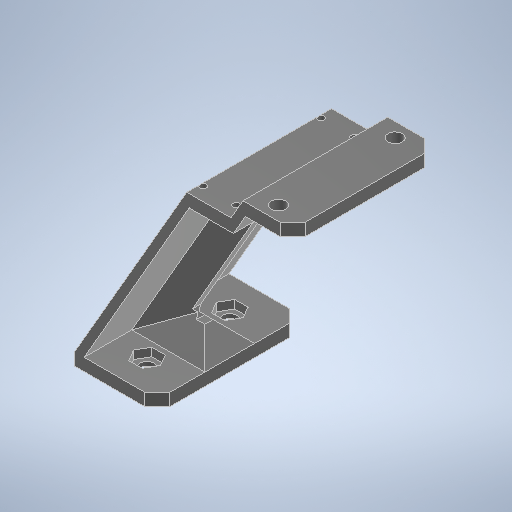
# Autodesk Inventor part: 3D_camera-fix
Saved by Autodesk Inventor 2025 (Build 290162000, 162)
## iProperties
Created: 2024-06-30
Part Number: 3D_camera-fix
Material: 一般
Document SubType Name: Modeling
Designer: 8326d
Density: 1 g/cm^3
Appearance: 滑らか - 黒
Author: 8326d
Autodesk Inventor part; units mm, degrees
ref_plane "YZ Plane" through (0, 0, 0) normal (1, 0, 0) x (0, 1, 0)
ref_plane "XZ Plane" through (0, 0, 0) normal (0, 1, 0) x (-1, 0, 0)
ref_plane "XY Plane" through (0, 0, 0) normal (0, 0, 1) x (1, 0, 0)
sketch "スケッチ1" plane through (0, 0, 0) normal (0, 0, 1) x (1, 0, 0)
  line L0 (120.5, 0) -> (-120.5, 0) construction
  line L1 (120.5, 0) -> (361.5, 0) construction
  line L2 (-120.5, 0) -> (-100.5, 0)
  line L3 (-100.5, 0) -> (-100.5, 3)
  line L4 (-100.5, 3) -> (-120.5, 3)
  line L5 (-120.5, 3) -> (-120.5, 0)
  line L6 (-120.5, 3) -> (-90.5, 54.961524) construction
  line L7 (-120.5, 3) -> (-60.5, 3) construction
  line L8 (-79.8, 54.961524) -> (-67.8, 54.961524)
  line L9 (-67.8, 54.961524) -> (-67.8, 51.961524)
  line L10 (-67.8, 51.961524) -> (-79.8, 51.961524)
  line L11 (-79.8, 51.961524) -> (-79.8, 54.961524)
  line L12 (-118.190599, 3) -> (-89.92265, 51.961524) construction
  line L13 (-118.190599, 3) -> (-92.809401, 46.961524)
  line L14 (-92.809401, 46.961524) -> (-82.109401, 46.961524)
  line L15 (-82.109401, 46.961524) -> (-79.22265, 51.961524)
  line L16 (-79.8, 54.961524) -> (-82.686751, 49.961524)
  line L17 (-82.686751, 49.961524) -> (-93.386751, 49.961524)
  line L18 (-93.386751, 49.961524) -> (-120.5, 3)
  point P0 (0, 0)
  point P1 (0, 0)
  point P2 (-118.190599, 3)
  dimension "d0" = 241
  dimension "d1" = 180
  dimension "d2" = 20
  dimension "d3" = 3
  dimension "d4" = 60
  dimension "d5" = 60
  dimension "d6" = 12
  dimension "d7" = 3
  dimension "d8" = 2
  dimension "d72" = 2
  dimension "d74" = 3
  dimension "d75" = 40.7
  dimension "d89" = 5
  constraints: 38 end point, 8 parallel, 6 horizontal, 3 point on line, 2 collinear, 2 equal length, 2 perpendicular, 1 coincident, 1 horizontal alignment, 1 midpoint
  measures "d0" distance of L0.start L0.end
  measures "d1" angle of L0 L1
  measures "d2" distance of L4.end L3.end
  measures "d3" distance of L3.end L2.end
  measures "d4" distance of L6.end L4.end
  measures "d5" angle of L7 L6
  measures "d6" distance of L9.end L10.end
  measures "d7" distance of L8.end L9.end
  measures "d8" distance between parallel lines of L6 L12
  measures "d72" distance between parallel lines of L16 L15
  measures "d74" distance between parallel lines of L14 L17
  measures "d75" distance between parallel lines of L5 L11
  measures "d89" distance between parallel lines of L8 L17
extrude "押し出し1" add sketch "スケッチ1" along normal mid plane 35
sketch "スケッチ2" plane through (0, 0, 0) normal (0, 0, 1) x (1, 0, 0)
  line L0 (-100.5, 3) -> (-120.5, 3)
  line L1 (-100.5, 3) -> (-105.5, 8)
  line L2 (-105.5, 8) -> (-109.530345, 8)
  line L3 (-76.335898, 46.961524) -> (-72.8, 46.961524)
  line L4 (-72.8, 46.961524) -> (-67.8, 51.961524)
  line L5 (-79.22265, 51.961524) -> (-82.109401, 46.961524)
  line L6 (-82.109401, 46.961524) -> (-92.809401, 46.961524)
  line L7 (-92.809401, 46.961524) -> (-118.190599, 3)
  line L8 (-76.335898, 46.961524) -> (-79.22265, 41.961524)
  line L9 (-79.22265, 41.961524) -> (-89.92265, 41.961524)
  line L10 (-89.92265, 41.961524) -> (-109.530345, 8)
  line L11 (-67.8, 51.961524) -> (-79.22265, 51.961524)
  point P0 (0, 0)
  dimension "d13" = 5
  dimension "d14" = 45
  dimension "d76" = 5
  dimension "d77" = 45
  dimension "d78" = 5
  constraints: 14 end point, 1 horizontal, 1 parallel, 2 other
  measures "d13" distance between parallel lines of L0 L2
  measures "d14" angle of L0 L1
  measures "d76" distance between parallel lines of L11 L3
  measures "d77" angle of L11 L4
  measures "d78" distance between parallel lines of L5 L8
extrude "押し出し2" add sketch "スケッチ2" along normal mid plane 2
chamfer "面取り1" distance 5 angle 45 10 edges at (-109.3453, 3, 1) (-109.3453, 3, -1) (-73.5113, 51.9615, -1) (-73.5113, 51.9615, 1) (-80.666, 49.4615, -1) (-87.4594, 46.9615, -1) (-105.5, 24.9808, -1) (-80.666, 49.4615, 1) (-87.4594, 46.9615, 1) (-105.5, 24.9808, 1)
chamfer "面取り2" distance 2 angle 45 4 edges at (-109.5303, 8, 0) (-76.3359, 46.9615, 0) (-89.9226, 41.9615, 0) (-79.2226, 41.9615, 0)
sketch "スケッチ3" plane through (-120.5, 0, 17.5) normal (0, -1, 0) x (1, 0, 0)
  line L0 (10, -7.5) -> (10, -27.5) construction
  line L1 (10, -7.5) -> (30, -7.5) construction
  line L2 (0, -35) -> (0, 0) construction
  point P0 (120.5, -17.5)
  point P1 (10, -17.5)
  point P2 (0, -17.5)
  dimension "d24" = 20
  dimension "d25" = 90
  dimension "d26" = 10
  constraints: 4 end point, 2 midpoint, 1 horizontal, 1 horizontal alignment, 1 perpendicular, 1 vertical
  measures "d24" distance of L0.start L0.end
  measures "d25" angle of L0 L1
  measures "d26" distance between parallel lines of L2 L0
hole "穴1" at (-110.5, 0, 10) at (-110.5, 0, -10) direction (0, 1, 0) diameter 3.5 depth 4 tip angle 118
sketch "スケッチ4" plane through (-100.5, 3, 17.5) normal (0, 1, 0) x (1, 0, 0)
  circle A0 centre (-10, 27.5) radius 1.75
  circle A1 centre (-10, 7.5) radius 1.75
  line L0 (-6.766838, 7.5) -> (-8.383419, 4.7)
  line L1 (-8.383419, 4.7) -> (-11.616581, 4.7)
  line L2 (-11.616581, 4.7) -> (-13.233162, 7.5)
  line L3 (-13.233162, 7.5) -> (-11.616581, 10.3)
  line L4 (-11.616581, 10.3) -> (-8.383419, 10.3)
  line L5 (-8.383419, 10.3) -> (-6.766838, 7.5)
  line L6 (-6.766838, 27.5) -> (-8.383419, 24.7)
  line L7 (-8.383419, 24.7) -> (-11.616581, 24.7)
  line L8 (-11.616581, 24.7) -> (-13.233162, 27.5)
  line L9 (-13.233162, 27.5) -> (-11.616581, 30.3)
  line L10 (-11.616581, 30.3) -> (-8.383419, 30.3)
  line L11 (-8.383419, 30.3) -> (-6.766838, 27.5)
  point P0 (100.5, 17.5)
  point P1 (-11.75, 30)
  point P2 (-8.25, 30)
  point P3 (-8.25, 0)
  point P4 (-11.75, 0)
  dimension "d34" = 5.6
  dimension "d35" = 5.6
  constraints: 24 end point, 2 coincident, 2 horizontal alignment, 28 other
  measures "d34" distance between parallel lines of L7 L10
  measures "d35" distance between parallel lines of L4 L1
extrude "押し出し3" cut sketch "スケッチ4" against normal blind 2 contours A0 | A1 | L0 L1 L2 L3 L4 L5 | L6 L7 L8 L9 L10 L11
sketch "スケッチ5" plane through (-79.8, 54.961524, 17.5) normal (0, 1, 0) x (1, 0, 0)
  line L0 (5.2, 31.6) -> (5.2, 3.4) construction
  line L1 (5.2, 31.6) -> (33.4, 31.6) construction
  line L2 (12, 35) -> (12, 0) construction
  line L3 (0, 35) -> (0, 0) projected
  point P0 (79.8, 17.5)
  point P1 (5.2, 17.5)
  dimension "d38" = 28.2
  dimension "d39" = 90
  dimension "d90" = 5.2
  constraints: 4 end point, 1 horizontal, 1 horizontal alignment, 1 midpoint, 1 perpendicular, 1 vertical
  measures "d38" distance of L0.start L0.end
  measures "d39" angle of L0 L1
  measures "d90" distance between parallel lines of L3 L0
hole "穴2" at (-74.6, 54.961524, -14.1) at (-74.6, 54.961524, 14.1) direction (0, -1, 0) diameter 3.5 depth 8 tip angle 118
chamfer "面取り4" distance 3 angle 45 4 edges at (-67.8, 53.4615, -17.5) (-67.8, 53.4615, 17.5) (-100.5, 1.5, -17.5) (-100.5, 1.5, 17.5)
sketch "スケッチ10" plane through (-93.386751, 49.961524, 17.5) normal (0, 1, 0) x (1, 0, 0)
  line L0 (8.7, 31.75) -> (0.7, 31.75) construction
  line L1 (0.7, 31.75) -> (0.7, 3.25) construction
  line L2 (0.7, 3.25) -> (8.7, 3.25) construction
  line L3 (8.7, 3.25) -> (8.7, 31.75) construction
  line L4 (8.7, 31.75) -> (0.7, 3.25) construction
  line L5 (0.7, 31.75) -> (8.7, 3.25) construction
  line L6 (25.586751, 32) -> (25.586751, 3) construction
  line L7 (10.7, 35) -> (10.7, 0) construction
  point P0 (93.386751, 17.5)
  point P1 (4.7, 17.5)
  point P2 (25.586751, 17.5)
  dimension "d79" = 8
  dimension "d80" = 28.5
  dimension "d81" = 2
  constraints: 12 end point, 3 midpoint, 2 parallel, 1 horizontal, 1 horizontal alignment, 1 perpendicular
  measures "d79" distance of L2.end L1.end
  measures "d80" distance of L1.end L0.end
  measures "d81" distance between parallel lines of L7 L3
hole "穴4" at (-92.686751, 49.961524, -14.25) at (-84.686751, 49.961524, -14.25) at (-84.686751, 49.961524, 14.25) at (-92.686751, 49.961524, 14.25) direction (0, -1, 0) diameter 1.6 depth 8 tip angle 118
equation "\"d7\" = d3"
equation "\"d72\" = d8"
equation "\"d13\" = d76"
equation "\"d77\" = d14"
equation "\"d35\" = d34"
